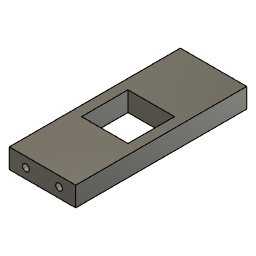
CameraHolder v13 (Autodesk Fusion 360 archive; units mm, degrees)
design "CameraHolder" references "tormach 770mx"
Autodesk Fusion 360 part; units mm, degrees
sketch "Sketch1" plane through (0, 0, 0) normal (0, 1, 0) x (1, 0, 0)
  line L0 (0, 0) -> (20, 0)
  line L1 (20, 0) -> (20, -51.54)
  line L2 (20, -51.54) -> (0, -51.54)
  line L3 (0, -51.54) -> (0, 0)
  dimension "d1" = 20
  dimension "d2" = 51.54
  constraint horizontal L0
  constraint vertical L1
  constraint horizontal L2
  constraint vertical L3
  constraint coincident L0.start L3.end
  measures "d1" distance of L0.start L0.end
  measures "d2" distance of L0.start L2.end
extrude "Extrude1" add sketch "Sketch1" along normal blind 5.92
sketch "Sketch2" plane through (0, 5.92, 0) normal (0, 1, 0) x (-1, 0, 0)
  line L0 (0, 51.54) -> (-20, 51.54)
  line L1 (-20, 51.54) -> (-20, 0)
  line L2 (-20, 0) -> (0, 0)
  line L3 (0, 0) -> (0, 51.54)
  line L4 (-10, 0) -> (-10, 49) construction
  line L5 (0, 25.77) -> (-20, 25.77) construction
  line L6 (-3, 32.77) -> (-17, 32.77)
  line L7 (-17, 32.77) -> (-17, 18.77)
  line L8 (-17, 18.77) -> (-3, 18.77)
  line L9 (-3, 18.77) -> (-3, 32.77)
  line L10 (-3, 32.77) -> (-17, 18.77) construction
  line L11 (-17, 32.77) -> (-3, 18.77) construction
  point P0 (-10, 25.77)
  dimension "d5" = 14
  dimension "d6" = 14
  constraint midpoint L2 L4.start
  constraint perpendicular L2 L4
  constraint midpoint L3 L5.start
  constraint midpoint L1 L5.end
  constraint horizontal L6
  constraint perpendicular L6 L7
  constraint parallel L6 L8
  constraint parallel L7 L9
  constraint coincident L10 P0
  constraint coincident L11 P0
  constraint midpoint L5 P0
  constraint coincident L9.start L8
  constraint coincident L8.end L9
  constraint coincident L7.end L8
  constraint coincident L8.start L7
  constraint coincident L6.start L9
  constraint coincident L9.end L6
  constraint coincident L6.end L7
  constraint coincident L7.start L6
  measures "d5" distance of L7.end L8.end
  measures "d6" distance of L6.end L7.end
extrude "Extrude2" cut sketch "Sketch2" along normal through all and the other way through all contours L6 L7 L8 L9
sketch "Sketch3" plane through (0, 0, 51.54) normal (0, 0, 1) x (1, 0, 0)
  line L0 (0, 0) -> (20, 0)
  line L1 (20, 0) -> (20, 5.92)
  line L2 (20, 5.92) -> (0, 5.92)
  line L3 (0, 5.92) -> (0, 0)
  line L4 (10, 5.92) -> (10, 0) construction
  line L5 (20, 2.96) -> (0, 2.96) construction
  point P0 (5, 2.96)
  point P1 (15, 2.96)
  dimension "d12" = 10
  dimension "d13" = 5
  constraint midpoint L2 L4.start
  constraint midpoint L0 L4.end
  constraint midpoint L1 L5.start
  constraint midpoint L3 L5.end
  constraint coincident L5 P0
  constraint coincident L5 P1
  measures "d12" distance of P0 P1
  measures "d13" distance of L5.end P0
hole "Hole1" at (5, 2.96, 51.54) direction (0, 0, -1) diameter 2.05 depth 10 tip angle 118
hole "Hole2" at (15, 2.96, 51.54) direction (0, 0, -1) diameter 2.05 depth 10 tip angle 118
sketch "Sketch4" plane through (0, 0, 0) normal (0, 0, -1) x (-1, 0, 0)
  line L0 (-20, 0) -> (0, 0)
  line L1 (0, 0) -> (0, 5.92)
  line L2 (0, 5.92) -> (-20, 5.92)
  line L3 (-20, 5.92) -> (-20, 0)
  line L4 (-20, 2.96) -> (0, 2.96) construction
  point P0 (-15, 2.96)
  point P1 (-5, 2.96)
  dimension "d30" = 10
  dimension "d31" = 5
  constraint midpoint L3 L4.start
  constraint midpoint L1 L4.end
  constraint coincident L4 P0
  constraint coincident L4 P1
  measures "d30" distance of P0 P1
  measures "d31" distance of L3 P0
hole "Hole5" at (15, 2.96, 0) direction (0, 0, 1) diameter 2.05 depth 10 tip angle 118
hole "Hole6" at (5, 2.96, 0) direction (0, 0, 1) diameter 2.05 depth 10 tip angle 118
